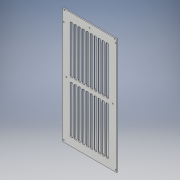
# Autodesk Inventor part: GlyphPlateUnderside
Saved by Autodesk Inventor 2017 (Build 210142000, 142)
## iProperties
Created: 2018-01-27
Part Number: GlyphPlateUnderside
Material: Generic
Document SubType Name: Modeling
Designer: User
Density: 1 g/cm^3
Appearance: Default
Author: User
Autodesk Inventor part; units mm, degrees
ref_plane "YZ Plane" through (0, 0, 0) normal (1, 0, 0) x (0, 1, 0)
ref_plane "XZ Plane" through (0, 0, 0) normal (0, 1, 0) x (-1, 0, 0)
ref_plane "XY Plane" through (0, 0, 0) normal (0, 0, 1) x (1, 0, 0)
sketch "Sketch1" plane through (0, 0, 0) normal (0, 0, 1) x (1, 0, 0)
  line L0 (0, 0) -> (178.2064, 0)
  line L1 (178.2064, 0) -> (178.2064, 381)
  line L2 (178.2064, 381) -> (0, 381)
  line L3 (0, 381) -> (0, 0)
  dimension "d0" = 178.2064
  dimension "d1" = 381
  constraints: 8 end point, 2 parallel, 1 horizontal, 1 perpendicular
  measures "d0" distance of L2.end L1.end
  measures "d1" distance of L1.end L0.end
extrude "Extrusion1" add sketch "Sketch1" along normal blind 3.175
sketch "Sketch2" plane through (0, 0, 3.175) normal (0, 0, 1) x (1, 0, 0)
  line L0 (0, 0) -> (178.2064, 0) projected
  line L1 (0, 0) -> (4.0386, 0)
  line L2 (4.0386, 0) -> (4.0386, 6.35)
  line L3 (0, 381) -> (0, 0) projected
  line L4 (0, 381) -> (4.0386, 381)
  line L5 (178.2064, 381) -> (0, 381) projected
  line L6 (4.0386, 381) -> (4.0386, 342.9)
  line L7 (4.0386, 381) -> (42.1386, 381) construction
  line L8 (0, 381) -> (0, 377.825)
  line L9 (0, 377.825) -> (6.35, 377.825)
  line L10 (178.2064, 0) -> (178.2064, 381) projected
  line L11 (178.2064, 0) -> (175.0314, 0)
  line L12 (175.0314, 0) -> (175.0314, 6.35)
  line L13 (178.2064, 377.825) -> (171.8564, 377.825)
  point P0 (175.0314, 368.3)
  dimension "d4" = 4.0386
  dimension "d5" = 6.35
  dimension "d6" = 38.1
  dimension "d7" = 90
  dimension "d8" = 3.175
  dimension "d9" = 6.35
  dimension "d10" = 3.175
  dimension "d11" = 6.35
  dimension "d19" = 4.0386
  dimension "d21" = 3.175
  dimension "d22" = 12.7
  dimension "d23" = 3.175
  constraints: 20 end point, 5 coincident, 5 perpendicular, 5 point on line, 1 horizontal, 1 vertical
  measures "d4" distance of L0.start L1.end
  measures "d5" distance of L1.end L2.end
  measures "d6" distance of L4.end L6.end
  measures "d7" angle of L6 L7
  measures "d8" distance of L3.start L8.end
  measures "d9" distance of L8.end L9.end
  measures "d10" distance of L0.end L11.end
  measures "d11" distance of L13.start L13.end
  measures "d19" distance between parallel lines of L3 L6
  measures "d21" distance from line of L10 point (175.031, 368.3)
  measures "d22" distance from line of point (175.031, 368.3) L5
  measures "d23" distance from line of L5 L13.end
hole "Hole1" at (4.0386, 6.35, 3.175) at (4.0386, 342.9, 3.175) at (6.35, 377.825, 3.175) at (175.0314, 6.35, 3.175) at (175.0314, 368.3, 3.175) at (171.8564, 377.825, 3.175) direction (0, 0, -1) diameter 3.556 depth 25.4 tip angle 118
sketch "Sketch3" plane through (0, 0, 3.175) normal (0, 0, 1) x (1, 0, 0)
  line L0 (30.1625, 25.4) -> (30.1625, 184.15) construction
  line L1 (34.925, 30.1625) -> (34.925, 179.3875)
  line L2 (25.4, 179.3875) -> (25.4, 30.1625)
  arc A0 (25.4, 30.1625) -> (34.925, 30.1625) centre (30.1625, 30.1625) ccw
  arc A1 (34.925, 179.3875) -> (25.4, 179.3875) centre (30.1625, 179.3875) ccw
  line L3 (0, 381) -> (0, 0) projected
  line L4 (0, 0) -> (178.2064, 0) projected
  line L5 (0, 381) -> (0, 0) projected
  line L6 (0, 190.5) -> (178.2064, 190.5)
  line L7 (43.2604, 25.4) -> (43.2604, 184.15) construction
  line L8 (48.0229, 30.1625) -> (48.0229, 179.3875)
  line L9 (38.4979, 179.3875) -> (38.4979, 30.1625)
  arc A2 (38.4979, 30.1625) -> (48.0229, 30.1625) centre (43.2604, 30.1625) ccw
  arc A3 (48.0229, 179.3875) -> (38.4979, 179.3875) centre (43.2604, 179.3875) ccw
  line L10 (56.3584, 25.4) -> (56.3584, 184.15) construction
  line L11 (61.1209, 30.1625) -> (61.1209, 179.3875)
  line L12 (51.5959, 179.3875) -> (51.5959, 30.1625)
  arc A4 (51.5959, 30.1625) -> (61.1209, 30.1625) centre (56.3584, 30.1625) ccw
  arc A5 (61.1209, 179.3875) -> (51.5959, 179.3875) centre (56.3584, 179.3875) ccw
  line L13 (69.4563, 25.4) -> (69.4563, 184.15) construction
  line L14 (74.2188, 30.1625) -> (74.2188, 179.3875)
  line L15 (64.6938, 179.3875) -> (64.6938, 30.1625)
  arc A6 (64.6938, 30.1625) -> (74.2188, 30.1625) centre (69.4563, 30.1625) ccw
  arc A7 (74.2188, 179.3875) -> (64.6938, 179.3875) centre (69.4563, 179.3875) ccw
  line L16 (82.5542, 25.4) -> (82.5542, 184.15) construction
  line L17 (87.3167, 30.1625) -> (87.3167, 179.3875)
  line L18 (77.7917, 179.3875) -> (77.7917, 30.1625)
  arc A8 (77.7917, 30.1625) -> (87.3167, 30.1625) centre (82.5542, 30.1625) ccw
  arc A9 (87.3167, 179.3875) -> (77.7917, 179.3875) centre (82.5542, 179.3875) ccw
  line L19 (95.6522, 25.4) -> (95.6522, 184.15) construction
  line L20 (100.4147, 30.1625) -> (100.4147, 179.3875)
  line L21 (90.8897, 179.3875) -> (90.8897, 30.1625)
  arc A10 (90.8897, 30.1625) -> (100.4147, 30.1625) centre (95.6522, 30.1625) ccw
  arc A11 (100.4147, 179.3875) -> (90.8897, 179.3875) centre (95.6522, 179.3875) ccw
  line L22 (108.7501, 25.4) -> (108.7501, 184.15) construction
  line L23 (113.5126, 30.1625) -> (113.5126, 179.3875)
  line L24 (103.9876, 179.3875) -> (103.9876, 30.1625)
  arc A12 (103.9876, 30.1625) -> (113.5126, 30.1625) centre (108.7501, 30.1625) ccw
  arc A13 (113.5126, 179.3875) -> (103.9876, 179.3875) centre (108.7501, 179.3875) ccw
  line L25 (121.848, 25.4) -> (121.848, 184.15) construction
  line L26 (126.6105, 30.1625) -> (126.6105, 179.3875)
  line L27 (117.0855, 179.3875) -> (117.0855, 30.1625)
  arc A14 (117.0855, 30.1625) -> (126.6105, 30.1625) centre (121.848, 30.1625) ccw
  arc A15 (126.6105, 179.3875) -> (117.0855, 179.3875) centre (121.848, 179.3875) ccw
  line L28 (134.946, 25.4) -> (134.946, 184.15) construction
  line L29 (139.7085, 30.1625) -> (139.7085, 179.3875)
  line L30 (130.1835, 179.3875) -> (130.1835, 30.1625)
  arc A16 (130.1835, 30.1625) -> (139.7085, 30.1625) centre (134.946, 30.1625) ccw
  arc A17 (139.7085, 179.3875) -> (130.1835, 179.3875) centre (134.946, 179.3875) ccw
  line L31 (148.0439, 25.4) -> (148.0439, 184.15) construction
  line L32 (152.8064, 30.1625) -> (152.8064, 179.3875)
  line L33 (143.2814, 179.3875) -> (143.2814, 30.1625)
  arc A18 (143.2814, 30.1625) -> (152.8064, 30.1625) centre (148.0439, 30.1625) ccw
  arc A19 (152.8064, 179.3875) -> (143.2814, 179.3875) centre (148.0439, 179.3875) ccw
  line L34 (178.2064, 0) -> (178.2064, 381) projected
  line L35 (30.1625, 355.6) -> (30.1625, 196.85) construction
  line L36 (34.925, 350.8375) -> (34.925, 201.6125)
  line L37 (25.4, 201.6125) -> (25.4, 350.8375)
  arc A20 (34.925, 350.8375) -> (25.4, 350.8375) centre (30.1625, 350.8375) ccw
  arc A21 (25.4, 201.6125) -> (34.925, 201.6125) centre (30.1625, 201.6125) ccw
  line L38 (43.2604, 355.6) -> (43.2604, 196.85) construction
  line L39 (48.0229, 350.8375) -> (48.0229, 201.6125)
  line L40 (38.4979, 201.6125) -> (38.4979, 350.8375)
  arc A22 (48.0229, 350.8375) -> (38.4979, 350.8375) centre (43.2604, 350.8375) ccw
  arc A23 (38.4979, 201.6125) -> (48.0229, 201.6125) centre (43.2604, 201.6125) ccw
  line L41 (56.3584, 355.6) -> (56.3584, 196.85) construction
  line L42 (61.1209, 350.8375) -> (61.1209, 201.6125)
  line L43 (51.5959, 201.6125) -> (51.5959, 350.8375)
  arc A24 (61.1209, 350.8375) -> (51.5959, 350.8375) centre (56.3584, 350.8375) ccw
  arc A25 (51.5959, 201.6125) -> (61.1209, 201.6125) centre (56.3584, 201.6125) ccw
  line L44 (69.4563, 355.6) -> (69.4563, 196.85) construction
  line L45 (74.2188, 350.8375) -> (74.2188, 201.6125)
  line L46 (64.6938, 201.6125) -> (64.6938, 350.8375)
  arc A26 (74.2188, 350.8375) -> (64.6938, 350.8375) centre (69.4563, 350.8375) ccw
  arc A27 (64.6938, 201.6125) -> (74.2188, 201.6125) centre (69.4563, 201.6125) ccw
  line L47 (82.5542, 355.6) -> (82.5542, 196.85) construction
  line L48 (87.3167, 350.8375) -> (87.3167, 201.6125)
  line L49 (77.7917, 201.6125) -> (77.7917, 350.8375)
  arc A28 (87.3167, 350.8375) -> (77.7917, 350.8375) centre (82.5542, 350.8375) ccw
  arc A29 (77.7917, 201.6125) -> (87.3167, 201.6125) centre (82.5542, 201.6125) ccw
  line L50 (95.6522, 355.6) -> (95.6522, 196.85) construction
  line L51 (100.4147, 350.8375) -> (100.4147, 201.6125)
  line L52 (90.8897, 201.6125) -> (90.8897, 350.8375)
  arc A30 (100.4147, 350.8375) -> (90.8897, 350.8375) centre (95.6522, 350.8375) ccw
  arc A31 (90.8897, 201.6125) -> (100.4147, 201.6125) centre (95.6522, 201.6125) ccw
  line L53 (108.7501, 355.6) -> (108.7501, 196.85) construction
  line L54 (113.5126, 350.8375) -> (113.5126, 201.6125)
  line L55 (103.9876, 201.6125) -> (103.9876, 350.8375)
  arc A32 (113.5126, 350.8375) -> (103.9876, 350.8375) centre (108.7501, 350.8375) ccw
  arc A33 (103.9876, 201.6125) -> (113.5126, 201.6125) centre (108.7501, 201.6125) ccw
  line L56 (121.848, 355.6) -> (121.848, 196.85) construction
  line L57 (126.6105, 350.8375) -> (126.6105, 201.6125)
  line L58 (117.0855, 201.6125) -> (117.0855, 350.8375)
  arc A34 (126.6105, 350.8375) -> (117.0855, 350.8375) centre (121.848, 350.8375) ccw
  arc A35 (117.0855, 201.6125) -> (126.6105, 201.6125) centre (121.848, 201.6125) ccw
  line L59 (134.946, 355.6) -> (134.946, 196.85) construction
  line L60 (139.7085, 350.8375) -> (139.7085, 201.6125)
  line L61 (130.1835, 201.6125) -> (130.1835, 350.8375)
  arc A36 (139.7085, 350.8375) -> (130.1835, 350.8375) centre (134.946, 350.8375) ccw
  arc A37 (130.1835, 201.6125) -> (139.7085, 201.6125) centre (134.946, 201.6125) ccw
  line L62 (148.0439, 355.6) -> (148.0439, 196.85) construction
  line L63 (152.8064, 350.8375) -> (152.8064, 201.6125)
  line L64 (143.2814, 201.6125) -> (143.2814, 350.8375)
  arc A38 (152.8064, 350.8375) -> (143.2814, 350.8375) centre (148.0439, 350.8375) ccw
  arc A39 (143.2814, 201.6125) -> (152.8064, 201.6125) centre (148.0439, 201.6125) ccw
  point P0 (30.1625, 104.775)
  point P1 (43.2604, 104.775)
  point P2 (56.3584, 104.775)
  point P3 (69.4563, 104.775)
  point P4 (82.5542, 104.775)
  point P5 (95.6522, 104.775)
  point P6 (108.7501, 104.775)
  point P7 (121.848, 104.775)
  point P8 (134.946, 104.775)
  point P9 (148.0439, 104.775)
  point P10 (30.1625, 276.225)
  point P11 (43.2604, 276.225)
  point P12 (56.3584, 276.225)
  point P13 (69.4563, 276.225)
  point P14 (82.5542, 276.225)
  point P15 (95.6522, 276.225)
  point P16 (108.7501, 276.225)
  point P17 (121.848, 276.225)
  point P18 (134.946, 276.225)
  point P19 (148.0439, 276.225)
  dimension "d27" = 25.4
  dimension "d34" = 25.4
  dimension "d39" = 381
  dimension "d53" = 190.5
  dimension "d54" = 6.35
  dimension "d57" = 13.0979
  dimension "d62" = 9.525
  dimension "d63" = 132.3181
  dimension "d64" = 127.4064
  dimension "d65" = 25.4
  constraints: 162 end point, 120 point on circle, 90 symmetric about line, 40 centre point, 40 point on line, 4 tangent, 2 midpoint, 1 horizontal, 1 parallel, 1 perpendicular, 1 vertical, 146 other
  measures "d27" distance between parallel lines of L3 L2
  measures "d34" distance from line of L4 L0.start
  measures "d39" distance of L4.end L34.end
  measures "d53" distance between parallel lines of L4 L6
  measures "d54" distance from line of L6 L0.end
  measures "d57" distance of L1.start L8.start
  measures "d62" distance between parallel lines of L2 L1
  measures "d64" distance between parallel lines of L32 L2
  measures "d65" distance between parallel lines of L34 L32
extrude "Extrusion2" cut sketch "Sketch3" against normal through all contours A0 L2 A1 L1 | A2 L9 A3 L8 | A4 L12 A5 L11 | A6 L15 A7 L14 | A8 L18 A9 L17 | A10 L21 A11 L20 | A12 L24 A13 L23 | A14 L27 A15 L26 | A16 L30 A17 L29 | A18 L33 A19 L32 | L36 A21 L37 A20 | L39 A23 L40 A22 | L42 A25 L43 A24 | L45 A27 L46 A26 | L48 A29 L49 A28 | L51 A31 L52 A30 | L54 A33 L55 A32 | L57 A35 L58 A34 | L60 A37 L61 A36 | L63 A39 L64 A38
sketch "Sketch4" plane through (0, 0, 3.175) normal (0, 0, 1) x (1, 0, 0)
  line L0 (178.2064, 381) -> (0, 381) projected
  line L1 (0, 381) -> (0, 0) projected
  line L2 (178.2064, 0) -> (178.2064, 381) projected
  line L3 (0, 0) -> (178.2064, 0) projected
  line L4 (25.4, 30.1625) -> (25.4, 179.3875) projected
  line L5 (152.8064, 179.3875) -> (152.8064, 30.1625) projected
  point P0 (12.7, 190.5)
  point P1 (165.5064, 190.5)
  point P2 (89.1032, 368.3)
  dimension "d68" = 381
  dimension "d69" = 190.5
  dimension "d70" = 190.5
  dimension "d71" = 25.4
  dimension "d72" = 12.7
  dimension "d73" = 12.7
  dimension "d74" = 178.2064
  dimension "d75" = 12.7
  dimension "d76" = 89.1032
  measures "d68" distance of L2.start L0.start
  measures "d69" distance from line of L3 point (165.506, 190.5)
  measures "d70" distance from line of L3 point (12.7, 190.5)
  measures "d71" distance between parallel lines of L1 L4
  measures "d72" distance from line of L1 point (12.7, 190.5)
  measures "d73" distance from line of point (165.506, 190.5) L2
  measures "d74" distance of L0.start L0.end
  measures "d75" distance from line of L0 point (89.103, 368.3)
  measures "d76" distance from line of L2 point (89.103, 368.3)
hole "Hole2" at (12.7, 190.5, 3.175) at (165.5064, 190.5, 3.175) at (89.1032, 368.3, 3.175) direction (0, 0, -1) diameter 3.556 end through all
equation "\"d34\" = d27"
equation "\"d53\" = 0.5 * d39"
equation "\"d57\" = -2.66667 * d64 + 2.66667 * d63"
equation "\"d65\" = d34"
equation "\"d69\" = 0.5 * d68"
equation "\"d70\" = d69"
equation "\"d72\" = 0.5 * d71"
equation "\"d73\" = d72"
equation "\"d75\" = d73"
equation "\"d76\" = 0.5 * d74"
body "Solid1"
